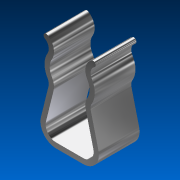
# Autodesk Inventor part: Soanar Power Module Fuse Holder
Saved by Autodesk Inventor 2016 (Build 200138000, 138)
## iProperties
Created: 2013-08-06
Material: Nickel-Copper Alloy 400
Document SubType Name: Modeling
Designer: sdarley
Density: 8.83 g/cm^3
Appearance: Chrome - Polished
Project: Power Entry Module - Soanar PP4003
Description: Soanar Power Module Fuse Holder
Author: sdarley
Title: Soanar Power Module Fuse Holder
Revision Number: 1
Autodesk Inventor part; units mm, degrees
ref_plane "YZ Plane" through (0, 0, 0) normal (1, 0, 0) x (0, 1, 0)
ref_plane "XZ Plane" through (0, 0, 0) normal (0, 1, 0) x (-1, 0, 0)
ref_plane "XY Plane" through (0, 0, 0) normal (0, 0, 1) x (1, 0, 0)
sketch "Sketch1" plane through (0, 0, 0) normal (0, 0, 1) x (1, 0, 0)
  line L0 (0, 0) -> (1.3, 0)
  line L1 (2.7559, 1.8612) -> (2.0235, 4.8129)
  arc A0 (1.3, 0) -> (2.7559, 1.8612) centre (1.3, 1.5) ccw
  arc A1 (2.1156, 5.4199) -> (2.0235, 4.8129) centre (2.8, 5.0056) ccw
  arc A2 (2.1156, 5.4199) -> (2.1156, 7.4913) centre (0.4047, 6.4556) ccw
  arc A3 (2.381, 8.587) -> (2.1156, 7.4913) centre (2.8, 7.9056) ccw
  arc A4 (2.381, 8.587) -> (2.119, 9.013) centre (2.25, 8.8) ccw
  arc A5 (2.119, 9.013) -> (1.6879, 7.2324) centre (2.8, 7.9056) ccw
  arc A6 (1.6879, 5.6788) -> (1.6879, 7.2324) centre (0.4047, 6.4556) ccw
  arc A7 (1.6879, 5.6788) -> (1.5383, 4.6925) centre (2.8, 5.0056) ccw
  arc A8 (1.3, 0.5) -> (2.2706, 1.7408) centre (1.3, 1.5) ccw
  line L2 (1.5383, 4.6925) -> (2.2706, 1.7408)
  line L3 (1.3, 0.5) -> (0, 0.5)
  line L4 (0, 0.5) -> (0, 0)
  point P0 (0, 0)
  dimension "d0" = 9.05
  dimension "d1" = 0.5
  dimension "d2" = 1.5
  dimension "d3" = 1.5
  dimension "d4" = 2.5
  dimension "d5" = 2.8
  dimension "d6" = 2.9
  dimension "d9" = 1.5
  dimension "d10" = 1.3
  dimension "d11" = 2
  constraints: 19 point on circle, 12 tangent, 10 end point, 9 centre point, 5 coincident, 2 parallel, 1 equal radius, 1 horizontal, 1 perpendicular
  measures "d1" distance between parallel lines of L0 L3
  measures "d2" distance edge to line of A7 L4
  measures "d3" distance edge to line of A5 L4
  measures "d6" distance of A1.centre A3.centre
  measures "d9" radius of A0
  measures "d10" radius of A7
  measures "d11" radius of A2
extrude "Extrusion1" add sketch "Sketch1" along normal mid plane 3.9
mirror "Mirror1" about plane through (0, 0, 0) normal (1, 0, 0) of "Extrusion1"
equation "\"d3\" = d2"
body "Solid1"
